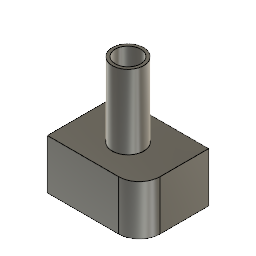
3.6 - presspull (Autodesk Fusion 360 design; units mm, degrees)
Autodesk Fusion 360 part; units mm, degrees
sketch "Sketch1" plane through (0, 0, 0) normal (0, 0, 1) x (1, 0, 0)
  line L0 (0, 0) -> (45.9912, 0)
  line L1 (45.9912, 0) -> (45.9912, 34.6951)
  line L2 (45.9912, 34.6951) -> (0, 34.6951)
  line L3 (0, 34.6951) -> (0, 0)
  circle A0 centre (22.9956, 17.3476) radius 7.8928
extrude "Extrude1" add sketch "Sketch1" against normal blind 24.87 contours L0 L1 L2 L3 | A0
extrude "Extrude2" add sketch "Sketch1" along normal blind 36.956 contours A0
fillet "Fillet1" radius 10.316 1 edges at (45.9912, 0, -12.435)
shell "Shell1" thickness 1.528 removed faces 1 at (18.3486, 16.3767, 36.956)
